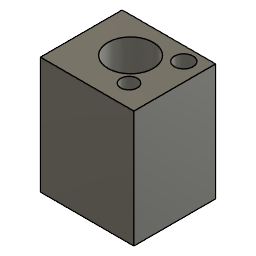
restu miling (Autodesk Fusion 360 design; units mm, degrees)
part number: 2026-06-24-22-19-34-982
Autodesk Fusion 360 part; units mm, degrees
sketch "Sketch1" plane through (0, 0, 0) normal (0, 1, 0) x (1, 0, 0)
  line L0 (0, 0) -> (80, 0)
  line L1 (80, 0) -> (80, 70)
  line L2 (80, 70) -> (0, 70)
  line L3 (0, 70) -> (0, 0)
  constraint horizontal L0
  constraint vertical L1
  constraint horizontal L2
  constraint vertical L3
  constraint coincident L0.start L3.end
extrude "Extrude1" add sketch "Sketch1" along normal blind 100
sketch "Sketch2" plane through (0, 100, 0) normal (0, 1, 0) x (-1, 0, 0)
  line L0 (0, -70) -> (0, 0)
  line L1 (0, 0) -> (-80, 0)
  line L2 (-80, 0) -> (-80, -70)
  line L3 (-80, -70) -> (0, -70)
  circle A0 centre (-37.2994, -39.884) radius 19.3144
  circle A1 centre (-57.1694, -18.6818) radius 7.126
  circle A2 centre (-64.4958, -58.2) radius 7.9468
extrude "Extrude2" cut sketch "Sketch2" against normal blind 50 contours A0 | A1 | A2
